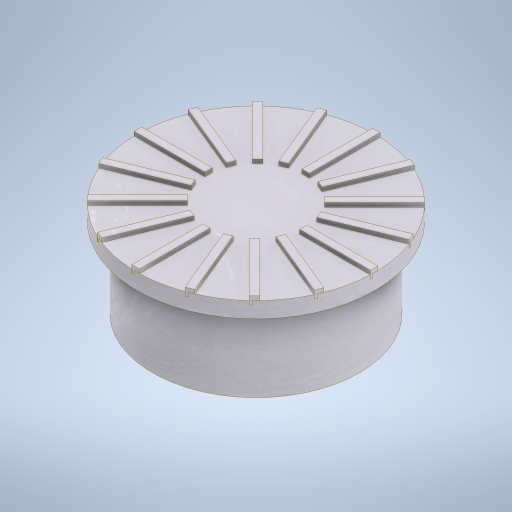
# Autodesk Inventor part: 圓
Saved by Autodesk Inventor 2024.2 (Build 282272000, 272)
## iProperties
Created: 2024-06-02
Part Number: 圓
Material: 一般
Document SubType Name: Modeling
Designer: sohil
Density: 1 g/cm^3
Appearance: 銀色
Author: sohil
Autodesk Inventor part; units mm, degrees
ref_plane "YZ Plane" through (0, 0, 0) normal (1, 0, 0) x (0, 1, 0)
ref_plane "XZ Plane" through (0, 0, 0) normal (0, 1, 0) x (-1, 0, 0)
ref_plane "XY Plane" through (0, 0, 0) normal (0, 0, 1) x (1, 0, 0)
sketch "草圖1" plane through (0, 0, 0) normal (0, 1, 0) x (-1, 0, 0)
  circle A0 centre (0, 0) radius 13
  dimension "d6" = 26
  constraints: 1 centre point
  measures "d6" diameter of A0
extrude "擠出1" add sketch "草圖1" along normal blind 10
sketch "草圖2" plane through (0, 10, 0) normal (0, 1, 0) x (1, 0, 0)
  circle A0 centre (0, 0) radius 15
  circle A1 centre (0, 0) radius 6.896935
  dimension "d9" = 30
  constraints: 2 centre point, 2 coincident
  measures "d9" diameter of A0
extrude "擠出2" add sketch "草圖2" along normal blind 2 contours A0 | A1
sketch "草圖3" plane through (0, 12, 0) normal (0, 1, 0) x (1, 0, 0)
  circle A0 centre (0, 0) radius 13
  circle A1 centre (0, 0) radius 15
  line L0 (-14.996254, -0.335194) -> (-6.102988, -0.335194)
  line L1 (-6.102988, -0.335194) -> (-6.102988, 0.610546)
  line L2 (-6.102988, 0.610546) -> (-14.996254, 0.610546)
  line L3 (-14.996254, 0.610546) -> (-14.996254, -0.335194)
  line L4 (-13.726459, -6.048497) -> (-5.510153, -2.645191)
  line L5 (-5.510153, -2.645191) -> (-5.872071, -1.771442)
  line L6 (-14.088378, -5.174747) -> (-13.726459, -6.048497)
  line L7 (-5.872071, -1.771442) -> (-14.088378, -5.174747)
  line L8 (-10.366935, -10.840971) -> (-4.078446, -4.552482)
  line L9 (-4.078446, -4.552482) -> (-4.747185, -3.883743)
  line L10 (-11.035674, -10.172232) -> (-10.366935, -10.840971)
  line L11 (-4.747185, -3.883743) -> (-11.035674, -10.172232)
  line L12 (-5.429139, -13.983006) -> (-2.025834, -5.766699)
  line L13 (-2.025834, -5.766699) -> (-2.899583, -5.40478)
  line L14 (-6.302889, -13.621087) -> (-5.429139, -13.983006)
  line L15 (-2.899583, -5.40478) -> (-6.302889, -13.621087)
  line L16 (0.335194, -14.996254) -> (0.335194, -6.102988)
  line L17 (0.335194, -6.102988) -> (-0.610546, -6.102988)
  line L18 (-0.610546, -14.996254) -> (0.335194, -14.996254)
  line L19 (-0.610546, -6.102988) -> (-0.610546, -14.996254)
  line L20 (6.048497, -13.726459) -> (2.645191, -5.510153)
  line L21 (2.645191, -5.510153) -> (1.771442, -5.872071)
  line L22 (5.174747, -14.088378) -> (6.048497, -13.726459)
  line L23 (1.771442, -5.872071) -> (5.174747, -14.088378)
  line L24 (10.840971, -10.366935) -> (4.552482, -4.078446)
  line L25 (4.552482, -4.078446) -> (3.883743, -4.747185)
  line L26 (10.172232, -11.035674) -> (10.840971, -10.366935)
  line L27 (3.883743, -4.747185) -> (10.172232, -11.035674)
  line L28 (13.983006, -5.429139) -> (5.766699, -2.025834)
  line L29 (5.766699, -2.025834) -> (5.40478, -2.899583)
  line L30 (13.621087, -6.302889) -> (13.983006, -5.429139)
  line L31 (5.40478, -2.899583) -> (13.621087, -6.302889)
  line L32 (14.996254, 0.335194) -> (6.102988, 0.335194)
  line L33 (6.102988, 0.335194) -> (6.102988, -0.610546)
  line L34 (14.996254, -0.610546) -> (14.996254, 0.335194)
  line L35 (6.102988, -0.610546) -> (14.996254, -0.610546)
  line L36 (13.726459, 6.048497) -> (5.510153, 2.645191)
  line L37 (5.510153, 2.645191) -> (5.872071, 1.771442)
  line L38 (14.088378, 5.174747) -> (13.726459, 6.048497)
  line L39 (5.872071, 1.771442) -> (14.088378, 5.174747)
  line L40 (10.366935, 10.840971) -> (4.078446, 4.552482)
  line L41 (4.078446, 4.552482) -> (4.747185, 3.883743)
  line L42 (11.035674, 10.172232) -> (10.366935, 10.840971)
  line L43 (4.747185, 3.883743) -> (11.035674, 10.172232)
  line L44 (5.429139, 13.983006) -> (2.025834, 5.766699)
  line L45 (2.025834, 5.766699) -> (2.899583, 5.40478)
  line L46 (6.302889, 13.621087) -> (5.429139, 13.983006)
  line L47 (2.899583, 5.40478) -> (6.302889, 13.621087)
  line L48 (-0.335194, 14.996254) -> (-0.335194, 6.102988)
  line L49 (-0.335194, 6.102988) -> (0.610546, 6.102988)
  line L50 (0.610546, 14.996254) -> (-0.335194, 14.996254)
  line L51 (0.610546, 6.102988) -> (0.610546, 14.996254)
  line L52 (-6.048497, 13.726459) -> (-2.645191, 5.510153)
  line L53 (-2.645191, 5.510153) -> (-1.771442, 5.872071)
  line L54 (-5.174747, 14.088378) -> (-6.048497, 13.726459)
  line L55 (-1.771442, 5.872071) -> (-5.174747, 14.088378)
  line L56 (-10.840971, 10.366935) -> (-4.552482, 4.078446)
  line L57 (-4.552482, 4.078446) -> (-3.883743, 4.747185)
  line L58 (-10.172232, 11.035674) -> (-10.840971, 10.366935)
  line L59 (-3.883743, 4.747185) -> (-10.172232, 11.035674)
  line L60 (-13.983006, 5.429139) -> (-5.766699, 2.025834)
  line L61 (-5.766699, 2.025834) -> (-5.40478, 2.899583)
  line L62 (-13.621087, 6.302889) -> (-13.983006, 5.429139)
  line L63 (-5.40478, 2.899583) -> (-13.621087, 6.302889)
  dimension "d12" = 360
  constraints: 128 end point, 2 parallel, 1 horizontal, 1 perpendicular, 131 other
sketch "草圖3 outline for 擠出3" plane through (0, 12, 0) normal (0, 1, 0) x (1, 0, 0)
  line L0 (6.102988, 0.335194) -> (6.102988, -0.610546)
  line L1 (14.996254, 0.335194) -> (6.102988, 0.335194)
  line L2 (14.996254, -0.610546) -> (14.996254, 0.335194)
  line L3 (6.102988, -0.610546) -> (14.996254, -0.610546)
  line L4 (5.766699, -2.025834) -> (5.40478, -2.899583)
  line L5 (13.983006, -5.429139) -> (5.766699, -2.025834)
  line L6 (13.621087, -6.302889) -> (13.983006, -5.429139)
  line L7 (5.40478, -2.899583) -> (13.621087, -6.302889)
  line L8 (4.552482, -4.078446) -> (3.883743, -4.747185)
  line L9 (10.840971, -10.366935) -> (4.552482, -4.078446)
  line L10 (10.172232, -11.035674) -> (10.840971, -10.366935)
  line L11 (3.883743, -4.747185) -> (10.172232, -11.035674)
  line L12 (2.645191, -5.510153) -> (1.771442, -5.872071)
  line L13 (6.048497, -13.726459) -> (2.645191, -5.510153)
  line L14 (5.174747, -14.088378) -> (6.048497, -13.726459)
  line L15 (1.771442, -5.872071) -> (5.174747, -14.088378)
  line L16 (0.335194, -6.102988) -> (-0.610546, -6.102988)
  line L17 (0.335194, -14.996254) -> (0.335194, -6.102988)
  line L18 (-0.610546, -14.996254) -> (0.335194, -14.996254)
  line L19 (-0.610546, -6.102988) -> (-0.610546, -14.996254)
  line L20 (-2.025834, -5.766699) -> (-2.899583, -5.40478)
  line L21 (-5.429139, -13.983006) -> (-2.025834, -5.766699)
  line L22 (-6.302889, -13.621087) -> (-5.429139, -13.983006)
  line L23 (-2.899583, -5.40478) -> (-6.302889, -13.621087)
  line L24 (-4.078446, -4.552482) -> (-4.747185, -3.883743)
  line L25 (-10.366935, -10.840971) -> (-4.078446, -4.552482)
  line L26 (-11.035674, -10.172232) -> (-10.366935, -10.840971)
  line L27 (-4.747185, -3.883743) -> (-11.035674, -10.172232)
  line L28 (-5.510153, -2.645191) -> (-5.872071, -1.771442)
  line L29 (-13.726459, -6.048497) -> (-5.510153, -2.645191)
  line L30 (-14.088378, -5.174747) -> (-13.726459, -6.048497)
  line L31 (-5.872071, -1.771442) -> (-14.088378, -5.174747)
  line L32 (-14.996254, 0.610546) -> (-14.996254, -0.335194)
  line L33 (-6.102988, 0.610546) -> (-14.996254, 0.610546)
  line L34 (-6.102988, -0.335194) -> (-6.102988, 0.610546)
  line L35 (-14.996254, -0.335194) -> (-6.102988, -0.335194)
  line L36 (-5.766699, 2.025834) -> (-5.40478, 2.899583)
  line L37 (-13.983006, 5.429139) -> (-5.766699, 2.025834)
  line L38 (-13.621087, 6.302889) -> (-13.983006, 5.429139)
  line L39 (-5.40478, 2.899583) -> (-13.621087, 6.302889)
  line L40 (-4.552482, 4.078446) -> (-3.883743, 4.747185)
  line L41 (-10.840971, 10.366935) -> (-4.552482, 4.078446)
  line L42 (-10.172232, 11.035674) -> (-10.840971, 10.366935)
  line L43 (-3.883743, 4.747185) -> (-10.172232, 11.035674)
  line L44 (-2.645191, 5.510153) -> (-1.771442, 5.872071)
  line L45 (-6.048497, 13.726459) -> (-2.645191, 5.510153)
  line L46 (-5.174747, 14.088378) -> (-6.048497, 13.726459)
  line L47 (-1.771442, 5.872071) -> (-5.174747, 14.088378)
  line L48 (-0.335194, 6.102988) -> (0.610546, 6.102988)
  line L49 (-0.335194, 14.996254) -> (-0.335194, 6.102988)
  line L50 (0.610546, 14.996254) -> (-0.335194, 14.996254)
  line L51 (0.610546, 6.102988) -> (0.610546, 14.996254)
  line L52 (2.025834, 5.766699) -> (2.899583, 5.40478)
  line L53 (5.429139, 13.983006) -> (2.025834, 5.766699)
  line L54 (6.302889, 13.621087) -> (5.429139, 13.983006)
  line L55 (2.899583, 5.40478) -> (6.302889, 13.621087)
  line L56 (5.510153, 2.645191) -> (5.872071, 1.771442)
  line L57 (13.726459, 6.048497) -> (5.510153, 2.645191)
  line L58 (14.088378, 5.174747) -> (13.726459, 6.048497)
  line L59 (5.872071, 1.771442) -> (14.088378, 5.174747)
  line L60 (4.078446, 4.552482) -> (4.747185, 3.883743)
  line L61 (10.366935, 10.840971) -> (4.078446, 4.552482)
  line L62 (11.035674, 10.172232) -> (10.366935, 10.840971)
  line L63 (4.747185, 3.883743) -> (11.035674, 10.172232)
extrude "擠出3" add sketch "草圖3 outline for 擠出3" along normal mid plane 1
